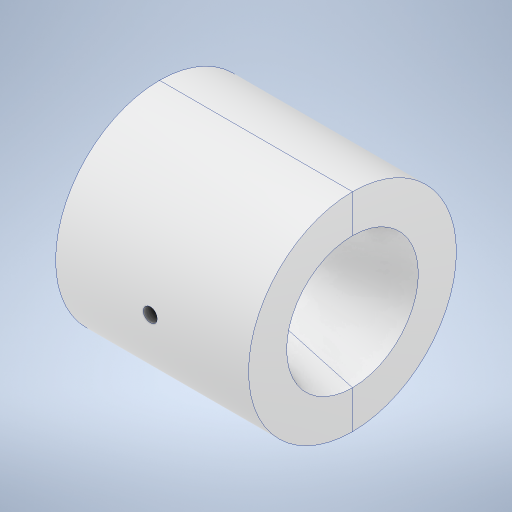
# Autodesk Inventor part: stainless steel space
Saved by Autodesk Inventor 2023 (Build 270158000, 158)
## iProperties
Created: 2022-09-19
Part Number: stainless steel space
Material: Aluminum 6061
Document SubType Name: Modeling
Designer: station
Density: 2.7 g/cm^3
Appearance: Aluminum - Flat
Author: station
Autodesk Inventor part; units mm, degrees
ref_plane "YZ Plane" through (0, 0, 0) normal (1, 0, 0) x (0, 1, 0)
ref_plane "XZ Plane" through (0, 0, 0) normal (0, 1, 0) x (-1, 0, 0)
sketch "Sketch3" plane through (0, 0, 0) normal (0, 0, 1) x (1, 0, 0)
  line L0 (254.7886, 18.124) -> (254.7886, 0) construction
  line L1 (192, 54.375) -> (254.7886, 18.124)
  line L2 (0, 0) -> (487.78, 0)
  line L3 (254.7886, 18.124) -> (256.7886, 18.124)
  line L4 (256.7886, 18.124) -> (327.1228, 36.97)
  line L5 (327.1228, 36.97) -> (327.1228, 0)
  line L6 (327.1228, 40.0758) -> (255.8936, 20.258)
  line L7 (255.8936, 20.258) -> (255.0924, 20.258)
  line L8 (255.0924, 20.258) -> (192.3194, 56.5)
  line L9 (327.1228, 36.97) -> (327.1228, 40.0758)
  line L10 (192, 54.375) -> (191.7835, 54.5)
  line L11 (0, 0) -> (0, 54.5)
  line L12 (0, 54.5) -> (274.8621, 54.5) construction
  line L13 (191.7835, 54.5) -> (188.7835, 54.5)
  line L14 (188.7835, 54.5) -> (188.7835, 56.5)
  line L15 (188.7835, 56.5) -> (192.3194, 56.5)
  line L16 (327.1228, 0) -> (327.1228, 59.5)
  line L17 (327.1228, 59.5) -> (323.1228, 59.5)
  line L18 (323.1228, 59.5) -> (323.1228, 38.9629)
  line L19 (323.1228, 59.5) -> (156.7613, 59.5)
  line L20 (323.1228, 59.5) -> (321.1228, 59.5)
  line L21 (321.1228, 59.5) -> (307.4068, 59.5)
  line L22 (255.7622, 23.3354) -> (330.1228, 44.0245)
  line L23 (185.7835, 59.5) -> (193.1232, 59.5)
  line L24 (196.9292, 57.3027) -> (255.7622, 23.3354)
  line L25 (307.4068, 59.5) -> (307.4068, 37.7043)
  line L26 (327.1228, 0) -> (251.1228, 0)
  line L27 (251.1228, 0) -> (251.1228, 85.8664)
  line L28 (196.9292, 59.5) -> (196.9292, 57.3027)
  point P0 (322.4487, 38.7754)
  point P1 (191.9595, 55.4142)
  point P2 (188.9595, 55.4)
  dimension "d65" = 18.124
  dimension "d66" = 30
  dimension "d67" = 18.124
  dimension "d68" = 2
  dimension "d69" = 15
  dimension "d70" = 36.97
  dimension "d71" = 2
  dimension "d72" = 54.5
  dimension "d73" = 3
  dimension "d74" = 2
  dimension "d75" = 59.5
  dimension "d76" = 4
  dimension "d77" = 2
  dimension "d78" = 13.716
  dimension "d79" = 3
  dimension "d90" = 76
  constraints: 58 end point, 11 point on line, 7 perpendicular, 4 vertical, 3 horizontal, 1 parallel
  measures "d65" distance of L0.start L0.end
  measures "d66" angle of L2 L1
  measures "d67" distance from line of L2 L0.start
  measures "d68" distance of L0.start L3.end
  measures "d69" angle of L2 L4
  measures "d70" distance of L4.end L5.end
  measures "d71" distance between parallel lines of L1 L8
  measures "d72" distance of L2.start L11.end
  measures "d73" distance of L10.end L13.end
  measures "d74" distance of L13.end L14.end
  measures "d75" distance of L5.end L16.end
  measures "d76" distance of L16.end L17.end
  measures "d77" distance of L17.end L20.end
  measures "d78" distance of L20.end L21.end
  measures "d79" distance between parallel lines of L6 L22
  measures "d90" distance of L5.end L26.end
revolve "Revolution2" add sketch "Sketch3" angle 360 about axis through (0, 0, 0) along (1, 0, 0) contours L27 L19 L25 L22 L24 | L24 L28 L19 L27
ref_plane "Work Plane2" through (0, 0, 59.5) normal (0, 0, 1) x (1, 0, 0)
sketch "Sketch5" plane through (0, 0, 59.5) normal (0, 0, 1) x (1, 0, 0)
  line L0 (307.4068, -37.7043) -> (307.4068, 37.7043) projected
  line L1 (307.4068, 0) -> (251.1228, 0) construction
  circle A0 centre (251.1228, 0) radius 4
  point P0 (0, 0)
  dimension "d91" = 56.284
  dimension "d92" = 8
  constraints: 2 end point, 1 centre point, 1 coincident, 1 horizontal, 1 midpoint
  measures "d91" distance of L1.start L1.end
  measures "d92" diameter of A0
extrude "Extrusion8" cut sketch "Sketch5" against normal blind 25
thread "Thread9" size "M8x1.25" class "6H" standard "ANSI Metric M Profile" full length
mirror "Mirror7" about plane through (0, 0, 0) normal (0, 0, 1) of "Extrusion8"
thread "Thread10" size "M8x1.25" class "6H" standard "ANSI Metric M Profile" full length
split_face "Split5"
body "Solid2"
